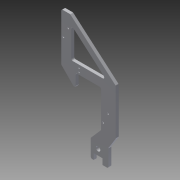
# Autodesk Inventor part: Rebuild Right Climber Hook
Saved by Autodesk Inventor 2014 SP1 (Build 180222100, 222)
## iProperties
Created: 2013-03-18
Part Number: Rebuild Right Climber Hook
Material: Aluminum 6061
Document SubType Name: Modeling
Designer: Arpan
Density: 2.71 g/cm^3
Mass: 180.618 g
Surface Area: 278.02 cm^2
Volume: 66.6486 cm^3
Appearance: Aluminum - Flat
Author: Arpan
Autodesk Inventor part; units mm, degrees
ref_plane "YZ Plane" through (0, 0, 0) normal (1, 0, 0) x (0, 1, 0)
sketch "Sketch1" plane through (0, 0, 0) normal (0, 0, 1) x (1, 0, 0)
  line L0 (0, 0) -> (6.35, 0)
  line L1 (6.35, 0) -> (6.35, 12.7)
  line L2 (6.35, 12.7) -> (25.4, 12.7)
  line L3 (25.4, 12.7) -> (25.4, 0)
  line L4 (25.4, 0) -> (31.75, 0)
  circle A0 centre (15.875, 25.4) radius 4.7816
  line L5 (-32.385, 142.875) -> (-32.385, 111.125)
  line L6 (-32.385, 142.875) -> (22.225, 142.875)
  line L7 (38.1, 38.1) -> (0, 38.1) construction
  line L8 (53.975, 0) -> (53.975, 161.925) construction
  line L9 (0, 38.1) -> (22.225, 63.5)
  line L10 (53.975, 63.5) -> (53.975, 161.925)
  line L11 (0, 0) -> (0, 38.1)
  line L12 (31.75, 0) -> (38.1, 0)
  line L13 (38.1, 0) -> (38.1, 38.1)
  line L14 (38.1, 38.1) -> (53.975, 63.5)
  line L15 (53.975, 63.5) -> (53.975, 161.925)
  line L16 (22.225, 63.5) -> (22.225, 142.875)
  line L17 (-32.385, 142.875) -> (22.225, 142.875)
  line L18 (0, 0) -> (0, 38.1)
  line L19 (0, 38.1) -> (22.225, 63.5)
  line L20 (22.225, 63.5) -> (22.225, 142.875)
  line L21 (22.225, 142.875) -> (-32.385, 142.875)
  line L22 (-32.385, 142.875) -> (-32.385, 111.125)
  line L23 (6.35, 12.7) -> (25.4, 12.7)
  line L24 (25.4, 12.7) -> (25.4, 0)
  line L25 (38.1, 0) -> (25.4, 0)
  line L26 (38.1, 0) -> (38.1, 38.1)
  line L27 (53.975, 63.5) -> (38.1, 38.1)
  line L28 (53.975, 63.5) -> (53.975, 161.925)
  line L29 (38.1, 0) -> (25.4, 0)
  line L30 (-63.5, 0) -> (-63.5, 246.5917) construction
  line L31 (-63.5, 142.875) -> (-63.5, 246.5917)
  line L32 (-63.5, 246.5917) -> (-44.45, 246.5917)
  line L33 (-32.385, 111.125) -> (-63.5, 142.875)
  line L34 (-44.45, 246.5917) -> (53.975, 161.925)
  line L35 (-41.91, 161.925) -> (34.5004, 161.925)
  line L36 (34.5004, 161.925) -> (-41.91, 227.6544)
  line L37 (-41.91, 161.925) -> (-41.91, 227.6544)
  dimension "d0" = 6.35
  dimension "d1" = 12.7
  dimension "d2" = 19.05
  dimension "d3" = 6.35
  dimension "d5" = 9.5631
  dimension "d6" = 12.7
  dimension "d7" = 9.525
  dimension "d11" = 31.75
  dimension "d23" = 25.4
  dimension "d24" = 38.1
  dimension "d25" = 25.4
  dimension "d26" = 38.1
  dimension "d27" = 54.61
  dimension "d32" = 6.35
  dimension "d33" = 22.225
  dimension "d34" = 38.1
  dimension "d36" = 79.375
  dimension "d60" = 117.475
  dimension "d61" = 103.7167
  dimension "d62" = 19.05
  dimension "d64" = 31.75
  dimension "d66" = 31.115
  dimension "d88" = 12.7
  dimension "d89" = 40.703
  dimension "d91" = 21.59
  dimension "d92" = 19.05
  constraints: 76 end point, 11 collinear, 8 perpendicular, 7 point on line, 4 horizontal, 4 parallel, 1 centre point, 1 vertical
  measures "d0" distance of L0.start L0.end
  measures "d1" distance of L0.end L1.end
  measures "d2" distance of L1.end L2.end
  measures "d3" distance of L3.end L4.end
  measures "d5" diameter of A0
  measures "d6" distance from line of L2 A0.centre
  measures "d7" distance from line of L1 A0.centre
  measures "d11" distance of L6.start L5.end
  measures "d23" vertical distance of L10.start L7.start
  measures "d24" distance from line of L4 L7.start
  measures "d25" vertical distance of L7.end L9.end
  measures "d26" distance of L0.start L7.end
  measures "d27" distance of L6.start L6.end
  measures "d32" distance of L4.end L12.end
  measures "d33" horizontal distance of L9.end L7.end
  measures "d34" distance of L7.end L13.end
  measures "d36" distance of L9.end L6.end
  measures "d60" distance between parallel lines of L30 L10
  measures "d61" distance of L31.start L31.end
  measures "d62" distance of L31.end L32.end
  measures "d64" vertical distance of L5.end L31.start
  measures "d66" distance from line of L5 L31.start
  measures "d88" distance between parallel lines of L36 L34
  measures "d89" angle of L35 L36
  measures "d91" distance from line of L30 L35.start
  measures "d92" distance from line of L6 L35.start
ref_plane "Work Plane1" through (0, 0, 9.525) normal (0, 0, 1) x (1, 0, 0)
ref_plane "Work Plane2" through (0, 0, 9.525) normal (0, 0, 1) x (1, 0, 0)
extrude "Extrusion6" add sketch "Sketch1" along normal blind 6.35
sketch "Sketch5" plane through (0, 0, 6.35) normal (0, 0, 1) x (1, 0, 0)
  line L0 (-44.45, 246.5917) -> (-63.5, 246.5917) projected
  line L1 (-63.5, 246.5917) -> (-63.5, 142.875) projected
  circle A0 centre (-48.755, 218.3215) radius 1.905
  circle A1 centre (-59.055, 196.6215) radius 1.905
  line L2 (-32.385, 142.875) -> (22.225, 142.875) projected
  line L3 (22.225, 142.875) -> (22.225, 63.5) projected
  circle A2 centre (36.97, 101.6) radius 1.905
  circle A3 centre (26.67, 79.9) radius 1.905
  dimension "d95" = 3.81
  dimension "d96" = 3.81
  dimension "d97" = 28.2702
  dimension "d99" = 4.445
  dimension "d123" = 10.3
  dimension "d124" = 21.7
  dimension "d125" = 3.81
  dimension "d126" = 3.81
  dimension "d127" = 10.3
  dimension "d128" = 21.7
  dimension "d129" = 41.275
  dimension "d130" = 4.445
  constraints: 4 centre point
  measures "d95" diameter of A0
  measures "d96" diameter of A1
  measures "d97" distance from line of L0 A0.centre
  measures "d99" distance from line of L1 A1.centre
  measures "d123" horizontal distance of A1.centre A0.centre
  measures "d124" vertical distance of A1.centre A0.centre
  measures "d125" diameter of A2
  measures "d126" diameter of A3
  measures "d127" horizontal distance of A3.centre A2.centre
  measures "d128" vertical distance of A3.centre A2.centre
  measures "d129" distance from line of L2 A2.centre
  measures "d130" distance from line of L3 A3.centre
extrude "Extrusion7" cut sketch "Sketch5" against normal blind 9.525
fillet "Fillet3" radius 3.175 16 edges at (-44.45, 246.5917, 3.175) (-63.5, 246.5917, 3.175) (53.975, 161.925, 3.175) (-41.91, 161.925, 3.175) (53.975, 63.5, 3.175) (38.1, 38.1, 3.175) (38.1, 0, 3.175) (0, 0, 3.175) (0, 38.1, 3.175) (22.225, 63.5, 3.175) (22.225, 142.875, 3.175) (-32.385, 111.125, 3.175) (-63.5, 142.875, 3.175) (-32.385, 142.875, 3.175) (-41.91, 227.6544, 3.175) (34.5004, 161.925, 3.175)
sketch "Sketch6" plane through (0, 0, 6.35) normal (0, 0, 1) x (1, 0, 0)
  line L0 (-29.21, 142.875) -> (19.05, 142.875) projected
  line L1 (25.9409, 161.925) -> (-38.735, 161.925) projected
  circle A0 centre (-25.4, 155.575) radius 1.5875
  circle A1 centre (-25.4, 147.6375) radius 1.5875
  line L2 (-63.5, 243.4167) -> (-63.5, 144.1714) projected
  point P0 (0, 0)
  dimension "d104" = 3.175
  dimension "d105" = 3.175
  dimension "d106" = 4.7625
  dimension "d107" = 6.35
  dimension "d110" = 38.1
  dimension "d111" = 38.1
  constraints: 2 centre point
  measures "d104" diameter of A0
  measures "d105" diameter of A1
  measures "d106" distance from line of L0 A1.centre
  measures "d107" distance from line of L1 A0.centre
  measures "d110" distance from line of A1.centre L2
  measures "d111" distance from line of L2 A0.centre
extrude "Extrusion8" cut sketch "Sketch6" against normal blind 9.525
sketch "Sketch7" plane through (0, 0, 6.35) normal (0, 0, 1) x (1, 0, 0)
  line L0 (-29.21, 142.875) -> (19.05, 142.875) projected
  line L1 (22.225, 139.7) -> (22.225, 64.693) projected
  line L2 (53.975, 104.775) -> (-210.9086, 104.775) construction
  circle A0 centre (38.354, 101.6) radius 1.905
  circle A1 centre (28.2448, 78.5876) radius 1.905
  line L3 (53.975, 64.4106) -> (53.975, 160.4681) projected
  point P0 (0, 0)
  dimension "d112" = 38.1
  dimension "d113" = 3.81
  dimension "d114" = 3.81
  dimension "d115" = 23.0124
  dimension "d116" = 10.1092
  dimension "d117" = 6.0198
  dimension "d118" = 3.175
  dimension "d121" = 264.8836
  constraints: 2 centre point, 2 end point, 1 point on line
  measures "d112" distance between parallel lines of L2 L0
  measures "d113" diameter of A0
  measures "d114" diameter of A1
  measures "d115" vertical distance of A1.centre A0.centre
  measures "d116" horizontal distance of A0.centre A1.centre
  measures "d117" distance from line of L1 A1.centre
  measures "d118" distance from line of L2 A0.centre
  measures "d121" distance of L2.start L2.end
extrude "Extrusion9" [suppressed]
body "Solid1"
